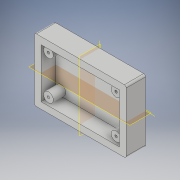
# Autodesk Inventor part: Case
Saved by Autodesk Inventor 2018 (Build 220112000, 112)
## iProperties
Created: 2018-09-30
Part Number: Case
Material: Generic
Document SubType Name: Modeling
Designer: andfro
Density: 1 g/cm^3
Appearance: Default
Author: andfro
Autodesk Inventor part; units mm, degrees
ref_plane "XY Plane" through (0, 0, 0) normal (0, 0, 1) x (1, 0, 0)
sketch "Sketch1" plane through (0, 0, 0) normal (0, 0, 1) x (1, 0, 0)
  line L0 (-47.5, -32.5) -> (47.5, -32.5)
  line L1 (47.5, -32.5) -> (47.5, 32.5)
  line L2 (47.5, 32.5) -> (-47.5, 32.5)
  line L3 (-47.5, 32.5) -> (-47.5, -32.5)
  point P0 (0, 0)
  point P1 (0, 32.5)
  point P2 (-47.5, 0)
  dimension "d0" = 65
  dimension "d1" = 95
  constraints: 8 end point, 2 midpoint, 2 parallel, 1 horizontal, 1 horizontal alignment, 1 perpendicular, 1 vertical alignment
  measures "d0" distance of L2.end L0.start
  measures "d1" distance of L1.end L2.end
extrude "Extrusion1" add sketch "Sketch1" along normal blind 20
sketch "Sketch4" plane through (0, 0, 20) normal (0, 0, 1) x (1, 0, 0)
  line L0 (-40.5, -25.7056) -> (40.5, -25.7056)
  line L1 (40.5, -25.7056) -> (40.5, 25.2944)
  line L2 (40.5, 25.2944) -> (-40.5, 25.2944)
  line L3 (-40.5, 25.2944) -> (-40.5, -25.7056)
  point P0 (0, 0)
  point P1 (0, 25.2944)
  point P2 (-40.5, -0.2056)
  dimension "d18" = 51
  dimension "d19" = 81
  constraints: 8 end point, 2 midpoint, 2 parallel, 1 horizontal, 1 perpendicular, 1 vertical alignment
  measures "d18" distance of L2.end L0.start
  measures "d19" distance of L1.end L2.end
extrude "Extrusion3" cut sketch "Sketch4" against normal blind 15
sketch "Sketch5" plane through (0, 0, 5) normal (0, 0, 1) x (1, 0, 0)
  circle A0 centre (-35, 20) radius 5
  point P0 (0, 0)
  dimension "d22" = 10
  dimension "d23" = 35
  dimension "d24" = 20
  constraints: 1 centre point
  measures "d22" diameter of A0
  measures "d23" horizontal distance of point (0, 0) A0.centre
  measures "d24" vertical distance of point (0, 0) A0.centre
extrude "Extrusion4" add sketch "Sketch5" along normal blind 13
sketch "Sketch6" plane through (-35, 20, 18) normal (0, 0, 1) x (1, 0, 0)
  circle A0 centre (0, 0) radius 5 projected
  point P0 (35, -20)
  constraints: 1 coincident
hole "Hole2" at (-35, 20, 18) direction (0, 0, -1) diameter 2.5 depth 8 tip angle 118
mirror "Mirror3" about plane through (0, 0, 0) normal (1, 0, 0) of "Extrusion4", "Hole2"
mirror "Mirror4" about plane through (0, 0, 0) normal (0, 1, 0) of "Extrusion4", "Hole2", "Mirror3"
fillet "Fillet1" radius 2 4 edges at (47.5, 32.5, 10) (47.5, -32.5, 10) (-47.5, -32.5, 10) (-47.5, 32.5, 10)
body "Solid1"
